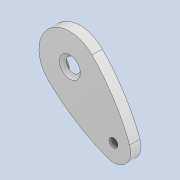
# Autodesk Inventor part: 原動節4v2
Saved by Autodesk Inventor 2020.4 (Build 244396000, 396)
## iProperties
Created: 2021-02-21
Part Number: 原動節4v2
Material: アルミニウム 2014-T4
Document SubType Name: Modeling
Designer: AA19065
Density: 2.8 g/cm^3
Appearance: サテン
Mass: 2.58269 g
Surface Area: 13.0506 cm^2
Volume: 0.922391 cm^3
Author: AA19065
Autodesk Inventor part; units mm, degrees
ref_plane "YZ Plane" through (0, 0, 0) normal (1, 0, 0) x (0, 1, 0)
ref_plane "XZ Plane" through (0, 0, 0) normal (0, 1, 0) x (-1, 0, 0)
ref_plane "XY Plane" through (0, 0, 0) normal (0, 0, 1) x (1, 0, 0)
sketch "スケッチ1" plane through (0, 0, 0) normal (0, 0, 1) x (1, 0, 0)
  arc A0 (-9.573129, 16.270325) -> (-8.082715, 13.688852) centre (-6.592301, 16.270325) ccw
  arc A1 (-7.527922, 12.727922) -> (-8.082715, 13.688852) centre (-8.637508, 12.727922) ccw
  arc A2 (-8.082715, 11.766993) -> (-7.527922, 12.727922) centre (-8.637508, 12.727922) ccw
  arc A3 (-8.082715, 11.766993) -> (-9.573129, 9.185519) centre (-6.592301, 9.185519) ccw
  arc A4 (-10.127922, 8.22459) -> (-9.573129, 9.185519) centre (-10.682715, 9.185519) ccw
  arc A5 (-11.237508, 8.22459) -> (-10.127922, 8.22459) centre (-10.682715, 9.185519) ccw
  arc A6 (-11.237508, 8.22459) -> (-14.218336, 8.22459) centre (-12.727922, 5.643117) ccw
  arc A7 (-15.327922, 8.22459) -> (-14.218336, 8.22459) centre (-14.773129, 9.185519) ccw
  arc A8 (-15.882715, 9.185519) -> (-15.327922, 8.22459) centre (-14.773129, 9.185519) ccw
  arc A9 (-15.882715, 9.185519) -> (-17.373129, 11.766993) centre (-18.863543, 9.185519) ccw
  arc A10 (-17.927922, 12.727922) -> (-17.373129, 11.766993) centre (-16.818336, 12.727922) ccw
  arc A11 (-17.373129, 13.688852) -> (-17.927922, 12.727922) centre (-16.818336, 12.727922) ccw
  arc A12 (-17.373129, 13.688852) -> (-15.882715, 16.270325) centre (-18.863543, 16.270325) ccw
  arc A13 (-15.327922, 17.231254) -> (-15.882715, 16.270325) centre (-14.773129, 16.270325) ccw
  arc A14 (-14.218336, 17.231254) -> (-15.327922, 17.231254) centre (-14.773129, 16.270325) ccw
  arc A15 (-14.218336, 17.231254) -> (-11.237508, 17.231254) centre (-12.727922, 19.812727) ccw
  arc A16 (-10.127922, 17.231254) -> (-11.237508, 17.231254) centre (-10.682715, 16.270325) ccw
  arc A17 (-9.573129, 16.270325) -> (-10.127922, 17.231254) centre (-10.682715, 16.270325) ccw
  circle A18 centre (-12.727922, 12.727922) radius 1.25
  circle A19 centre (-12.727922, 12.727922) radius 9
  circle A20 centre (0, 0) radius 1.25
  circle A21 centre (0, 0) radius 5
  arc A22 (-19.005066, 6.278313) -> (-1.763106, -4.678831) centre (15.867957, 42.109476) ccw
  arc A23 (4.678831, 1.763106) -> (-6.278313, 19.005066) centre (-42.109476, -15.867957) ccw
  dimension "d0" = 2.5
  dimension "d1" = 10
  dimension "d2" = 50
  constraints: 44 point on circle, 24 centre point, 4 tangent, 2 coincident, 1 equal radius, 21 other
  measures "d0" diameter of A20
  measures "d1" diameter of A21
  measures "d2" radius of A22
sketch "スケッチ1 outline for 押し出し1" plane through (0, 0, 0) normal (0, 0, 1) x (1, 0, 0)
  arc A0 (-6.278313, 19.005066) -> (-19.005066, 6.278313) centre (-12.727922, 12.727922) ccw
  arc A1 (4.678831, 1.763106) -> (-6.278313, 19.005066) centre (-42.109476, -15.867957) ccw
  arc A2 (-19.005066, 6.278313) -> (-1.763106, -4.678831) centre (15.867957, 42.109476) ccw
  arc A3 (-1.763106, -4.678831) -> (4.678831, 1.763106) centre (0, 0) ccw
  circle A4 centre (0, 0) radius 1.25
  circle A5 centre (-12.727922, 12.727922) radius 1.25
extrude "押し出し1" add sketch "スケッチ1 outline for 押し出し1" along normal blind 3
chamfer "面取り1" distance 1.8 angle 45 1 edges at (-13.9779, 12.7279, 3)
sketch "スケッチ1 outline for 押し出し3" plane through (0, 0, 0) normal (0, 0, 1) x (1, 0, 0)
  arc A0 (-14.218336, 17.231254) -> (-15.327922, 17.231254) centre (-14.773129, 16.270325) ccw
  arc A1 (-11.237508, 17.231254) -> (-14.218336, 17.231254) centre (-12.727922, 19.812727) cw
  arc A2 (-15.327922, 17.231254) -> (-15.882715, 16.270325) centre (-14.773129, 16.270325) ccw
  arc A3 (-10.127922, 17.231254) -> (-11.237508, 17.231254) centre (-10.682715, 16.270325) ccw
  arc A4 (-15.882715, 16.270325) -> (-17.373129, 13.688852) centre (-18.863543, 16.270325) cw
  arc A5 (-9.573129, 16.270325) -> (-10.127922, 17.231254) centre (-10.682715, 16.270325) ccw
  arc A6 (-17.373129, 13.688852) -> (-17.927922, 12.727922) centre (-16.818336, 12.727922) ccw
  arc A7 (-8.082715, 13.688852) -> (-9.573129, 16.270325) centre (-6.592301, 16.270325) cw
  arc A8 (-17.927922, 12.727922) -> (-17.373129, 11.766993) centre (-16.818336, 12.727922) ccw
  arc A9 (-7.527922, 12.727922) -> (-8.082715, 13.688852) centre (-8.637508, 12.727922) ccw
  arc A10 (-17.373129, 11.766993) -> (-15.882715, 9.185519) centre (-18.863543, 9.185519) cw
  arc A11 (-8.082715, 11.766993) -> (-7.527922, 12.727922) centre (-8.637508, 12.727922) ccw
  arc A12 (-15.882715, 9.185519) -> (-15.327922, 8.22459) centre (-14.773129, 9.185519) ccw
  arc A13 (-9.573129, 9.185519) -> (-8.082715, 11.766993) centre (-6.592301, 9.185519) cw
  arc A14 (-15.327922, 8.22459) -> (-14.218336, 8.22459) centre (-14.773129, 9.185519) ccw
  arc A15 (-10.127922, 8.22459) -> (-9.573129, 9.185519) centre (-10.682715, 9.185519) ccw
  arc A16 (-14.218336, 8.22459) -> (-11.237508, 8.22459) centre (-12.727922, 5.643117) cw
  arc A17 (-11.237508, 8.22459) -> (-10.127922, 8.22459) centre (-10.682715, 9.185519) ccw
  circle A18 centre (-12.727922, 12.727922) radius 1.25
extrude "押し出し3" cut sketch "スケッチ1 outline for 押し出し3" along normal blind 2
sketch "スケッチ2" plane through (0, 0, 0) normal (0, 0, -1) x (-1, 0, 0)
  arc A0 (11.237508, 17.231254) -> (14.218336, 17.231254) centre (12.727922, 19.812727) ccw
  arc A1 (15.882715, 16.270325) -> (14.218336, 17.231254) centre (14.773129, 16.270325) ccw
  arc A2 (15.882715, 16.270325) -> (17.373129, 13.688852) centre (18.863543, 16.270325) ccw
  arc A3 (17.373129, 11.766993) -> (17.373129, 13.688852) centre (16.818336, 12.727922) ccw
  arc A4 (17.373129, 11.766993) -> (15.882715, 9.185519) centre (18.863543, 9.185519) ccw
  arc A5 (14.218336, 8.22459) -> (15.882715, 9.185519) centre (14.773129, 9.185519) ccw
  arc A6 (14.218336, 8.22459) -> (11.237508, 8.22459) centre (12.727922, 5.643117) ccw
  arc A7 (9.573129, 9.185519) -> (11.237508, 8.22459) centre (10.682715, 9.185519) ccw
  arc A8 (9.573129, 9.185519) -> (8.082715, 11.766993) centre (6.592301, 9.185519) ccw
  arc A9 (8.082715, 13.688852) -> (8.082715, 11.766993) centre (8.637508, 12.727922) ccw
  arc A10 (8.082715, 13.688852) -> (9.573129, 16.270325) centre (6.592301, 16.270325) ccw
  arc A11 (11.237508, 17.231254) -> (9.573129, 16.270325) centre (10.682715, 16.270325) ccw
  arc A12 (1.763106, -4.678831) -> (19.005066, 6.278313) centre (-15.867957, 42.109476) ccw
  arc A13 (19.005066, 6.278313) -> (6.278313, 19.005066) centre (12.727922, 12.727922) ccw
  arc A14 (6.278313, 19.005066) -> (-4.678831, 1.763106) centre (42.109476, -15.867957) ccw
  arc A15 (-4.678831, 1.763106) -> (1.763106, -4.678831) centre (0, 0) ccw
  circle A16 centre (0, 0) radius 1.25
  circle A17 centre (12.727922, 12.727922) radius 7.5
  arc A18 (7.353248, 17.958876) -> (-3.275181, 1.234174) centre (42.109476, -15.867957) ccw
  arc A19 (17.958876, 7.353248) -> (7.353248, 17.958876) centre (12.727922, 12.727922) ccw
  arc A20 (1.234174, -3.275181) -> (17.958876, 7.353248) centre (-15.867957, 42.109476) ccw
  arc A21 (-3.275181, 1.234174) -> (1.234174, -3.275181) centre (0, 0) ccw
  circle A22 centre (12.727922, 12.727922) radius 2.05
  circle A23 centre (0, 0) radius 4
  line L0 (12.727922, 12.727922) -> (0, 0)
  line L1 (12.374369, 13.081475) -> (-0.353553, 0.353553)
  line L2 (13.081475, 12.374369) -> (0.353553, -0.353553)
  point P0 (7.789973, 7.082866)
  point P1 (3.159796, 2.45269)
  point P2 (3.100332, -2.527437)
  point P3 (17.958876, 7.353248)
  point P4 (2.45269, 3.159796)
  point P5 (7.082866, 7.789973)
  point P6 (7.353248, 17.958876)
  point P7 (-2.527437, 3.100332)
  dimension "d12" = 15
  dimension "d13" = 1.5
  dimension "d14" = 8
  dimension "d15" = 0.5
  dimension "d16" = 0.5
  constraints: 8 point on circle, 6 centre point, 6 end point, 2 parallel, 1 coincident, 1 concentric, 3 other
  measures "d12" diameter of A17
  measures "d13" radial gap between concentric circles of A14 A18
  measures "d14" diameter of A23
  measures "d15" distance between parallel lines of L0 L1
  measures "d16" distance between parallel lines of L0 L2
sketch "スケッチ2 outline for 押し出し4" plane through (0, 0, 0) normal (0, 0, -1) x (-1, 0, 0)
  arc A0 (17.958876, 7.353248) -> (7.353248, 17.958876) centre (12.727922, 12.727922) cw
  arc A1 (7.353248, 17.958876) -> (-2.527437, 3.100332) centre (42.109476, -15.867957) ccw
  arc A2 (-2.527437, 3.100332) -> (3.100332, -2.527437) centre (0, 0) cw
  arc A3 (3.100332, -2.527437) -> (17.958876, 7.353248) centre (-15.867957, 42.109476) ccw
extrude "押し出し4" cut sketch "スケッチ2 outline for 押し出し4" against normal blind 2.7
fillet "フィレット1" radius 2 4 edges at (-7.3532, 17.9589, 1.35) (-17.9589, 7.3532, 1.35) (2.5274, 3.1003, 1.35) (-3.1003, -2.5274, 1.35)
sketch "書き出し" plane through (0, 0, 0) normal (0, 0, -1) x (-1, 0, 0)
  arc A0 (5.505927, 10.704857) -> (10.704857, 5.505927) centre (12.727922, 12.727922) ccw
  arc A1 (11.285086, 1.922883) -> (10.704857, 5.505927) centre (10.165373, 3.580062) ccw
  arc A2 (6.848479, -0.741587) -> (11.285086, 1.922883) centre (-15.867957, 42.109476) ccw
  arc A3 (3.941146, 0.683645) -> (6.848479, -0.741587) centre (5.911719, 1.025467) ccw
  arc A4 (3.941146, 0.683645) -> (0.683645, 3.941146) centre (0, 0) ccw
  arc A5 (-0.741587, 6.848479) -> (0.683645, 3.941146) centre (1.025467, 5.911719) ccw
  arc A6 (1.922883, 11.285086) -> (-0.741587, 6.848479) centre (42.109476, -15.867957) ccw
  arc A7 (5.505927, 10.704857) -> (1.922883, 11.285086) centre (3.580062, 10.165373) ccw
  arc A8 (11.237508, 17.231254) -> (14.218336, 17.231254) centre (12.727922, 19.812727) ccw
  arc A9 (15.882715, 16.270325) -> (14.218336, 17.231254) centre (14.773129, 16.270325) ccw
  arc A10 (15.882715, 16.270325) -> (17.373129, 13.688852) centre (18.863543, 16.270325) ccw
  arc A11 (17.373129, 11.766993) -> (17.373129, 13.688852) centre (16.818336, 12.727922) ccw
  arc A12 (17.373129, 11.766993) -> (15.882715, 9.185519) centre (18.863543, 9.185519) ccw
  arc A13 (14.218336, 8.22459) -> (15.882715, 9.185519) centre (14.773129, 9.185519) ccw
  arc A14 (14.218336, 8.22459) -> (11.237508, 8.22459) centre (12.727922, 5.643117) ccw
  arc A15 (9.573129, 9.185519) -> (11.237508, 8.22459) centre (10.682715, 9.185519) ccw
  arc A16 (9.573129, 9.185519) -> (8.082715, 11.766993) centre (6.592301, 9.185519) ccw
  arc A17 (8.082715, 13.688852) -> (8.082715, 11.766993) centre (8.637508, 12.727922) ccw
  arc A18 (8.082715, 13.688852) -> (9.573129, 16.270325) centre (6.592301, 16.270325) ccw
  arc A19 (11.237508, 17.231254) -> (9.573129, 16.270325) centre (10.682715, 16.270325) ccw
  arc A20 (1.763106, -4.678831) -> (19.005066, 6.278313) centre (-15.867957, 42.109476) ccw
  arc A21 (19.005066, 6.278313) -> (6.278313, 19.005066) centre (12.727922, 12.727922) ccw
  arc A22 (6.278313, 19.005066) -> (-4.678831, 1.763106) centre (42.109476, -15.867957) ccw
  arc A23 (-4.678831, 1.763106) -> (1.763106, -4.678831) centre (0, 0) ccw
  circle A24 centre (0, 0) radius 1.25
  circle A25 centre (12.727922, 12.727922) radius 2.05
